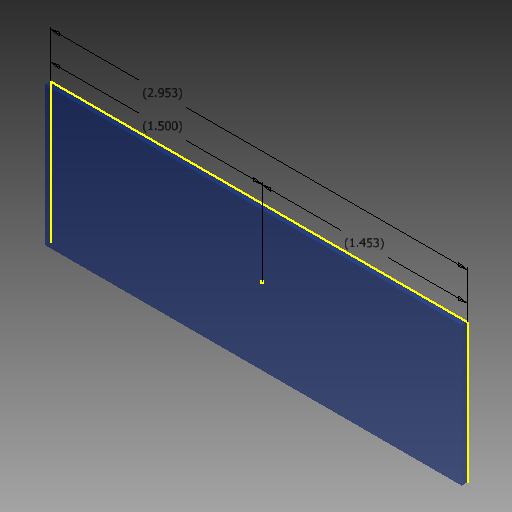
# Autodesk Inventor part: SLIDE - 25X75
Saved by Autodesk Inventor 2018.3 (Build 223284000, 284)
## iProperties
Created: 2010-10-27
Part Number: SLIDE - 25X75
Material: Glass
Document SubType Name: Modeling
Designer: COOPB
Mass: 4.28686 g
Surface Area: 40.7741 cm^2
Volume: 1.96645 cm^3
Density: 2.18 g/cm^3
Appearance: Blue (Clear)
Author: COOPB
Revision Number: 0
Autodesk Inventor part; units mm, degrees
ref_plane "YZ Plane" through (0, 0, 0) normal (1, 0, 0) x (0, 1, 0)
ref_plane "XZ Plane" through (0, 0, 0) normal (0, 1, 0) x (-1, 0, 0)
ref_plane "XY Plane" through (0, 0, 0) normal (0, 0, 1) x (1, 0, 0)
derived "JF-GM-VL-0041 SLIDE MOUNTING PLATE.ipt"
sketch "Sketch1" plane through (0, 0, 0) normal (0, 0, 1) x (1, 0, 0)
  line L0 (0, 62.23) -> (0, -62.23) construction
  line L1 (-63.4058, 0) -> (69.2849, 0) construction
  line L2 (-44.45, 44.45) -> (44.45, 44.45)
  line L3 (44.45, 44.45) -> (44.45, -44.45)
  line L4 (44.45, -44.45) -> (-44.45, -44.45)
  line L5 (-44.45, -44.45) -> (-44.45, 44.45)
  line L6 (31.75, 31.75) -> (-31.75, 31.75) construction
  line L7 (-31.75, 31.75) -> (-31.75, -31.75) construction
  line L8 (-31.75, -31.75) -> (31.75, -31.75) construction
  line L9 (31.75, -31.75) -> (31.75, 31.75) construction
  line L10 (-38.1, 14.224) -> (39.624, 14.224)
  line L11 (39.624, 14.224) -> (39.624, -12.7)
  line L12 (39.624, -12.7) -> (-38.1, -12.7)
  line L13 (-38.1, -12.7) -> (-38.1, 14.224)
  circle A0 centre (-38.1, 14.224) radius 3.302
  circle A1 centre (-38.1, -12.7) radius 3.302
  line L14 (-19.05, -13.208) -> (-19.05, -44.45)
  line L15 (-19.05, -44.45) -> (19.05, -44.45)
  line L16 (19.05, -44.45) -> (19.05, -13.208)
  line L17 (-12.7, 13.208) -> (-12.7, 20.574)
  arc A2 (-9.398, 23.876) -> (-12.7, 20.574) centre (-9.398, 20.574) ccw
  line L18 (-9.398, 23.876) -> (9.398, 23.876)
  arc A3 (12.7, 20.574) -> (9.398, 23.876) centre (9.398, 20.574) ccw
  line L19 (12.7, 20.574) -> (12.7, 13.208)
  line L20 (-9.398, 9.906) -> (9.398, 9.906)
  line L21 (-15.748, -9.906) -> (15.748, -9.906)
  arc A4 (-12.7, 13.208) -> (-9.398, 9.906) centre (-9.398, 13.208) ccw
  arc A5 (9.398, 9.906) -> (12.7, 13.208) centre (9.398, 13.208) ccw
  arc A6 (-15.748, -9.906) -> (-19.05, -13.208) centre (-15.748, -13.208) ccw
  arc A7 (19.05, -13.208) -> (15.748, -9.906) centre (15.748, -13.208) ccw
  line L22 (-38.1, -12.7) -> (38.1, -12.7)
  line L23 (38.1, -12.7) -> (38.1, 12.7)
  line L24 (38.1, 12.7) -> (-38.1, 12.7)
  line L25 (-38.1, 12.7) -> (-38.1, -12.7)
  line L26 (-38.1, -12.7) -> (38.1, 12.7) construction
  arc A8 (38.1, 12.7) -> (49.4215, 22.2135) centre (31.75, 31.75) ccw construction
  arc A9 (40.8788, 8.0472) -> (47.7671, 12.0368) centre (31.75, 31.75) ccw
  line L27 (47.7671, 12.0368) -> (38.8331, 34.5596)
  line L28 (28.7639, 18.6118) -> (26.4225, 24.5144)
  circle A10 centre (31.75, 31.75) radius 4.3656
  line L29 (31.75, 31.75) -> (35.9321, 21.2069) construction
  arc A11 (38.8331, 34.5596) -> (31.6627, 39.3695) centre (31.75, 31.75) ccw
  line L30 (31.6627, 39.3695) -> (-18.9391, 38.7898)
  arc A12 (-18.9391, 38.7898) -> (-19.4465, 32.487) centre (-18.9028, 35.6151) ccw
  line L31 (-19.4465, 32.487) -> (26.4225, 24.5144)
  line L32 (-18.9028, 35.6151) -> (31.75, 31.75) construction
  line L33 (31.75, 31.75) -> (26.4225, 24.5144) construction
  circle A13 centre (39.624, -12.7) radius 3.302
  line L34 (-7.1755, 27.1717) -> (-24.638, 28.6995)
  circle A14 centre (31.75, 31.75) radius 4.3148
  arc A15 (40.8788, 8.0472) -> (28.7639, 18.6118) centre (1.8543, -24.4755) ccw
  line L35 (39.624, 4.327) -> (44.45, 7.1133)
  line L36 (-24.638, 28.6995) -> (-24.638, 44.45)
  arc A16 (-16.1868, 37.8508) -> (-15.9605, 24.0774) centre (31.75, 31.75) ccw
  arc A17 (-21.1002, 38.4762) -> (-20.8507, 23.291) centre (31.75, 31.75) ccw
  arc A18 (-20.8507, 23.291) -> (-15.9605, 24.0774) centre (-18.4056, 23.6842) ccw
  arc A19 (-18.9028, 35.6151) -> (-18.4056, 23.6842) centre (31.75, 31.75) ccw construction
  circle A20 centre (-18.9028, 35.6151) radius 2.3813 construction
  line L37 (-19.006, 29.635) -> (-19.2777, 36.1557) construction
  circle A21 centre (-18.0554, 21.7467) radius 2.3749 construction
  line L38 (-18.0554, 21.7467) -> (-18.0912, 21.7395) construction
  arc A22 (-16.1868, 37.8508) -> (-21.1002, 38.4762) centre (-18.6435, 38.1635) ccw
  arc A23 (-7.3194, 23.876) -> (-7.1755, 27.1717) centre (-7.3194, 25.527) ccw
  line L39 (-7.3194, 23.876) -> (-7.3194, 4.327)
  line L40 (-7.3194, 4.327) -> (39.624, 4.327)
  line L41 (-38.1, 12.3) -> (36.9, 12.3)
  line L42 (36.9, 12.3) -> (36.9, -12.7)
  line L43 (-38.1, 12.3) -> (-38.1, -12.7)
  line L44 (-38.1, -12.7) -> (36.9, -12.7)
  point P0 (0, 31.75)
  point P1 (0, -31.75)
  point P2 (-31.75, 0)
  point P3 (31.75, 0)
extrude "Extrusion1" add sketch "Sketch1" along normal blind 1.016 contours A6 L21 A7 L12 | L12 A1 L13 A0 L41 A4 L20 L39 L40 L42 A13 A7 L21 A6 | L12 L13 A1 | A13 L42 L12 | L13 L41 A0 | L40 L39 L20 A5 L41 L42 | A5 L20 L39 L41 | L39 L20 A4 L41 picked at (-36.9362, -10.8478)
sketch "Sketch2" plane through (0, 0, 0) normal (0, 0, 1) x (1, 0, 0)
  line L0 (-38.1, -12.7) -> (-38.1, 12.3) projected
  line L1 (36.9, 12.3) -> (36.9, -12.7) projected
  line L2 (-38.1, 12.3) -> (36.9, 12.3) projected
  point P0 (0, 0)
  dimension "d3" = 75
  dimension "d4" = 38.1
  dimension "d5" = 36.9
  measures "d3" distance of L0.end L1.start
  measures "d4" distance from line of point (0, 0) L0
  measures "d5" distance from line of L1 point (0, 0)
body "Solid1"
